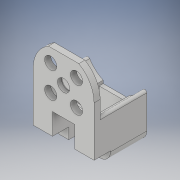
# Autodesk Inventor part: uchyt motoru-final
Saved by Autodesk Inventor 2018 (Build 220112000, 112)
## iProperties
Created: 2018-03-10
Part Number: uchyt motoru-final
Material: Všeobecné
Document SubType Name: Modeling
Designer: Kuba
Density: 1 g/cm^3
Appearance: Výchozí
Author: Kuba
Autodesk Inventor part; units mm, degrees
note: some values were not read from the file. Chosen so that the rebuilt part matches the saved one: sketch regions of "Vysunutí1".
sketch "Náčrt1" plane through (0, 0, 0) normal (0, 1, 0) x (-1, 0, 0)
  arc A0 (2.75, -6.9776) -> (-2.75, -6.9776) centre (0, 0) ccw
  line L0 (-7.5, 0) -> (-7.5, -15)
  line L1 (7.5, -15) -> (7.5, 0)
  line L2 (2.75, -6.9776) -> (-2.75, -6.9776)
  line L3 (-2.75, -6.9776) -> (-2.75, -15)
  line L4 (2.75, -15) -> (2.75, -6.9776)
  circle A1 centre (4.5, 0) radius 1.5
  circle A2 centre (0, 0) radius 1.5
  circle A3 centre (0, 4.5) radius 1.5
  circle A4 centre (-4.5, 0) radius 1.5
  circle A5 centre (0, -4.5) radius 1.5
  line L5 (-7.5, -15) -> (-2.75, -15)
  line L6 (2.75, -15) -> (7.5, -15)
  circle A6 centre (3.182, 3.182) radius 1.5
  circle A7 centre (0, 4.5) radius 1.5
  circle A8 centre (-3.182, 3.182) radius 1.5
  circle A9 centre (-4.5, 0) radius 1.5
  circle A10 centre (-3.182, -3.182) radius 1.5
  circle A11 centre (0, -4.5) radius 1.5
  circle A12 centre (3.182, -3.182) radius 1.5
  line L7 (-1.5, 0) -> (-3, 0)
  line L8 (-6, 0) -> (-7.5, 0)
  line L9 (7.5, 0) -> (6, 0)
  line L10 (3, 0) -> (1.5, 0)
  dimension "d0" = 15
  dimension "d1" = 3
  dimension "d2" = 3
  dimension "d5" = 360
  dimension "d7" = 4.5
  dimension "d8" = 5.5
  dimension "d9" = 15
  dimension "d10" = 15
  dimension "d13" = 360
  constraints: 22 end point, 13 centre point, 10 parallel, 9 point on circle, 5 horizontal, 5 perpendicular, 2 coincident, 26 other
  measures "d0" diameter of A0
  measures "d1" diameter of A1
  measures "d2" diameter of A2
  measures "d7" distance of point (0, 0) A1.centre
  measures "d8" distance of L2.start L2.end
  measures "d9" distance between parallel lines of L0 L1
  measures "d10" distance of L1.start L1.end
extrude "Vysunutí1" add sketch "Náčrt1" along normal blind 1.5 contours L2 A0 L8 A4 L7 A2 L10 A1 L9 | A0 L1 L6 L4 | L9 A1 L10 A2 L7 A4 L8 A0 | L3 L5 L0 A0 | A1 | A4 | A3 | A5
ref_plane "Pracovní rovina1" through (0, 1.5, 0) normal (0, 1, 0) x (1, 0, 0)
sketch "Náčrt3" plane through (0, 1.5, 0) normal (0, 1, 0) x (1, 0, 0)
  arc A0 (7.5, 1.9526) -> (-7.5, 1.9526) centre (0, 0) ccw
  line L0 (-7.5, 15) -> (-7.5, 0) projected
  line L1 (7.5, 15) -> (2.75, 15) projected
  line L2 (7.5, 1.9526) -> (7.5, 15)
  line L3 (7.5, 15) -> (-7.5, 15)
  line L4 (-7.5, 15) -> (-7.5, 1.9526)
  dimension "d18" = 15.5
  constraints: 6 end point, 2 point on circle, 1 centre point, 1 coincident, 1 parallel, 1 point on line
  measures "d18" diameter of A0
extrude "Vysunutí2" add sketch "Náčrt3" along normal blind 11.5
ref_plane "Pracovní rovina2" through (-2.75, 0, -15) normal (0, 0, -1) x (-1, 0, 0)
sketch "Náčrt4" plane through (-2.75, 0, -15) normal (0, 0, -1) x (-1, 0, 0)
  line L0 (-5.5, 0) -> (-5.5, 1.5) projected
  line L1 (-5.5, 1.5) -> (0, 1.5)
  line L2 (0, 1.5) -> (0, 4.5)
  line L3 (0, 4.5) -> (-5.5, 4.5)
  line L4 (-5.5, 4.5) -> (-5.5, 1.5)
  point P0 (-2.75, 0)
  dimension "d51" = 3
  constraints: 8 end point, 2 parallel, 1 horizontal, 1 perpendicular
  measures "d51" distance of L3.end L0.end
extrude "Vysunutí3" cut sketch "Náčrt4" against normal blind 9
fillet "Zaoblení1" radius 0.5 1 edges at (7.5, 7.25, -1.9526)
fillet "Zaoblení2" radius 0.5 1 edges at (-7.5, 7.25, -1.9526)
sketch "Náčrt9" plane through (-2.75, 0, -15) normal (0, 0, -1) x (-1, 0, 0)
  line L0 (0, 0) -> (0, 4.5) projected
  line L1 (0, 0) -> (4.75, 0) projected
  line L2 (4.75, 0) -> (4.75, 13) projected
  line L3 (-10.25, 13) -> (4.75, 13) projected
  line L4 (-10.25, 0) -> (-10.25, 13) projected
  line L5 (-10.25, 0) -> (-5.5, 0) projected
  line L6 (-5.5, 0) -> (-5.5, 4.5) projected
  line L7 (-6, 5.5) -> (0.5, 5.5)
  line L8 (0.5, 5.5) -> (0.5, 12)
  line L9 (0.5, 12) -> (-6, 12)
  line L10 (-6, 12) -> (-6, 5.5)
  line L11 (-5.5, 4.5) -> (0, 4.5) projected
  point P0 (-2.75, 0)
  dimension "d28" = 6.5
  dimension "d29" = 6.5
  dimension "d31" = 0.5
  dimension "d50" = 1
  constraints: 8 end point, 2 parallel, 1 horizontal, 1 perpendicular
  measures "d28" distance of L9.end L7.start
  measures "d29" distance of L8.end L9.end
  measures "d31" distance between parallel lines of L6 L10
  measures "d50" distance between parallel lines of L3 L9
extrude "Vysunutí5" cut sketch "Náčrt9" against normal blind 8 contours L10 L9 L8 L7
fillet "Zaoblení4" radius 0.5 1 edges at (1.5, 1.5, 0)
fillet "Zaoblení5" radius 2.5 2 edges at (-7.5, 6.5, -15) (7.5, 6.5, -15)
fillet "Zaoblení6" radius 0.5 2 edges at (0, 4.5, -7.75) (0, 1.5, -6.9776)
ref_plane "Pracovní rovina3" through (0, 13, 0) normal (0, 1, 0) x (1, 0, 0)
sketch "Náčrt10" plane through (0, 13, 0) normal (0, 1, 0) x (1, 0, 0)
  arc A0 (3.25, 7.0356) -> (-3.25, 7.0356) centre (0, 0) ccw projected
  line L0 (-3.25, 15) -> (-3.25, 7.0356) projected
  line L1 (3.25, 15) -> (-3.25, 15) projected
  line L2 (3.25, 15) -> (3.25, 7.0356) projected
  line L3 (3.25, 7.0356) -> (-3.25, 7.0356)
  line L4 (-3.25, 7.0356) -> (-3.25, 7.75)
  line L5 (-3.25, 7.75) -> (3.25, 7.75)
  line L6 (3.25, 7.75) -> (3.25, 7.0356)
  constraints: 8 end point, 2 parallel, 1 horizontal, 1 perpendicular, 1 point on line
extrude "Vysunutí6" cut sketch "Náčrt10" against normal blind 2 contours L3 A0 | A0 L5 L2 | A0 L0 L5
sketch "Sketch11" plane through (-7.5, 0, 0) normal (-1, 0, 0) x (0, 0, 1)
  line L0 (-15, 0) -> (-6.9776, 0) projected
  line L1 (-15, 0) -> (-12.25, 0)
  line L2 (-12.25, 0) -> (-12.25, 4)
  line L3 (-12.25, 4) -> (-15, 4)
  line L4 (-15, 4) -> (-15, 0)
  point P0 (0, 0)
  dimension "d42" = 2.75
  dimension "d43" = 4
  constraints: 8 end point, 2 parallel, 1 horizontal, 1 perpendicular
  measures "d42" distance of L3.end L2.end
  measures "d43" distance of L2.end L1.end
extrude "Extrusion7" cut sketch "Sketch11" against normal through all
sketch "Sketch12" plane through (0, 0, 0) normal (0, -1, 0) x (1, 0, 0)
  line L0 (7.5804, 6.5) -> (-7.5515, 6.5)
  line L1 (-7.5515, 6.5) -> (-7.5515, 9.7793)
  line L2 (-7.5515, 9.7793) -> (7.5804, 9.7793)
  line L3 (7.5804, 9.7793) -> (7.5804, 6.5)
  arc A0 (7.5, 0) -> (-7.5, 0) centre (0, 0) ccw projected
  dimension "d46" = 1
  constraints: 8 end point, 2 parallel, 1 horizontal, 1 perpendicular
  measures "d46" distance edge to line of A0 L0
extrude "Extrusion8" cut sketch "Sketch12" against normal through all
sketch "Sketch13" plane through (-2.75, 1.5, -7.2457) normal (1, 0, 0) x (0, 0, -1)
  line L0 (7.7543, 2.5) -> (7.7543, 3) projected
  line L1 (7.7543, 3) -> (3.5043, 3)
  line L2 (3.5043, 3) -> (3.5043, 4)
  line L3 (3.5043, 4) -> (7.7543, 4)
  line L4 (7.7543, 4) -> (7.7543, 3)
  line L5 (5.0043, -1.5) -> (5.0043, 2.5) projected
  point P0 (-7.2457, -1.5)
  dimension "d52" = 1.5
  constraints: 8 end point, 2 parallel, 1 horizontal, 1 perpendicular, 1 point on line
  measures "d52" distance from line of L1.end L5
extrude "Extrusion9" cut sketch "Sketch13" along normal up to surface (5.5 mm away)
fillet "Fillet8" radius 0.5 1 edges at (0, 4.5, -10.75)
equation "\"d9\" = d0"
equation "\"d29\" = d28"
equation "\"d31\" = -0.5 * d8 + 0.5 * d28"
